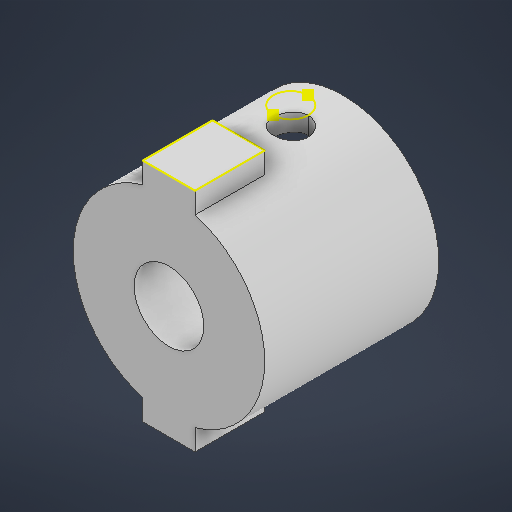
# Autodesk Inventor part: Wheel_Lego_Axle_Connector_2
Saved by Autodesk Inventor 2025 (Build 290162010, 162A)
## iProperties
Created: 2024-07-02
Part Number: Wheel_Lego_Axle_Connector_2
Material: Generic
Document SubType Name: Modeling
Designer: chaya
Density: 1 g/cm^3
Appearance: Default
Author: chaya
Autodesk Inventor part; units mm, degrees
ref_plane "YZ Plane" through (0, 0, 0) normal (1, 0, 0) x (0, 1, 0)
ref_plane "XZ Plane" through (0, 0, 0) normal (0, 1, 0) x (-1, 0, 0)
ref_plane "XY Plane" through (0, 0, 0) normal (0, 0, 1) x (1, 0, 0)
derived "Wheel_Lego_Axle_Connector.ipt"
sketch "Connector_Sketch" plane through (0, 0, 10) normal (0, 0, 1) x (1, 0, 0)
  line L0 (-1.5, -6.3246) -> (-1.5, -5.2915)
  arc A0 (-1.5, 5.2915) -> (-1.5, -5.2915) centre (0, 0) ccw
  line L1 (-1.5, 5.2915) -> (-1.5, 6.3246)
  arc A1 (-1.5, 6.3246) -> (-1.5, -6.3246) centre (0, 0) ccw
  line L2 (1.5, -5.2915) -> (1.5, -6.3246)
  arc A2 (1.5, -6.3246) -> (1.5, 6.3246) centre (0, 0) ccw
  line L3 (1.5, 6.3246) -> (1.5, 5.2915)
  arc A3 (1.5, -5.2915) -> (1.5, 5.2915) centre (0, 0) ccw
sketch "Connector_2_Sketch" plane through (0, 6.5, 0) normal (0, 1, 0) x (-1, 0, 0)
  line L0 (-1.5, 6) -> (1.5, 6)
  line L1 (1.5, 10) -> (1.5, 6)
  line L2 (-1.5, 6) -> (-1.5, 10)
  spline S0 degree 3 poles (0, 4) (0.1258, 4) (0.2598, 3.9748) (0.5061, 3.8727) (0.6184, 3.7958) (0.7958, 3.6184) (0.8727, 3.5061) (0.9748, 3.2598) (1, 3.1258) (1, 3) (1, 2.8742) (0.9748, 2.7402) (0.8727, 2.4939) (0.7958, 2.3816) (0.6184, 2.2042) (0.5061, 2.1273) (0.2598, 2.0252) (0.1258, 2) (0, 2) knots 0 0 0 0 0.124999 0.124999 0.249998 0.249998 0.374999 0.374999 0.5 0.5 0.5 0.625001 0.625001 0.750002 0.750002 0.875001 0.875001 1 1 1 1
  spline S1 degree 3 poles (0, 2) (-0.1258, 2) (-0.2598, 2.0252) (-0.5061, 2.1273) (-0.6184, 2.2042) (-0.7958, 2.3816) (-0.8727, 2.4939) (-0.9748, 2.7402) (-1, 2.8742) (-1, 3.1258) (-0.9748, 3.2598) (-0.8727, 3.5061) (-0.7958, 3.6184) (-0.6184, 3.7958) (-0.5061, 3.8727) (-0.2598, 3.9748) (-0.1258, 4) (0, 4) knots 0 0 0 0 0.124999 0.124999 0.249998 0.249998 0.374999 0.374999 0.5 0.5 0.625001 0.625001 0.750002 0.750002 0.875001 0.875001 1 1 1 1
  line L3 (1.5, 10) -> (-1.5, 10)
sketch "Connector_3_Sketch" plane through (0, -6.5, 0) normal (0, 1, 0) x (-1, 0, 0)
  line L0 (1.5, 10) -> (1.5, 6)
  line L1 (-1.5, 6) -> (1.5, 6)
  line L2 (-1.5, 10) -> (-1.5, 6)
  line L3 (1.5, 10) -> (1.5, 6)
  line L4 (1.5, 10) -> (-1.5, 10)
sketch "Sketch3" plane through (0, 0, 0) normal (0, 0, 1) x (1, 0, 0)
  arc A0 (1.5, -5.2915) -> (1.5, 5.2915) centre (0, 0) ccw construction
  arc A1 (-1.5, 5.2915) -> (-1.5, -5.2915) centre (0, 0) ccw construction
  circle A2 centre (0, 0) radius 5.5
  circle A3 centre (0, 0) radius 4.5
  dimension "d1" = 9
  constraints: 2 centre point, 2 coincident, 1 concentric
  measures "d1" diameter of A3
extrude "Extrusion1" add sketch "Sketch3" along normal blind 10
extrude "Extrusion3" cut sketch "Connector_2_Sketch" against normal through all contours S0 S1
extrude "Extrusion4" add sketch "Connector_2_Sketch" against normal up to surface contours L2 L3 L1 L0 round surface about axis through (0, 0, 0) along (0, 0, 1) radius 4.5 far side no
extrude "Extrusion5" add sketch "Connector_3_Sketch" along normal up to surface round surface about axis through (0, 0, 0) along (0, 0, 1) radius 4.5 far side no
sketch "Sketch6" plane through (0, 0, 10) normal (0, 0, 1) x (1, 0, 0)
  circle A0 centre (0, 0) radius 4.5 projected
  circle A1 centre (0, 0) radius 2
  dimension "d14" = 4
  constraints: 1 centre point, 1 coincident
  measures "d14" diameter of A1
extrude "Extrusion6" add sketch "Sketch6" against normal blind 3
body "Solid1"
